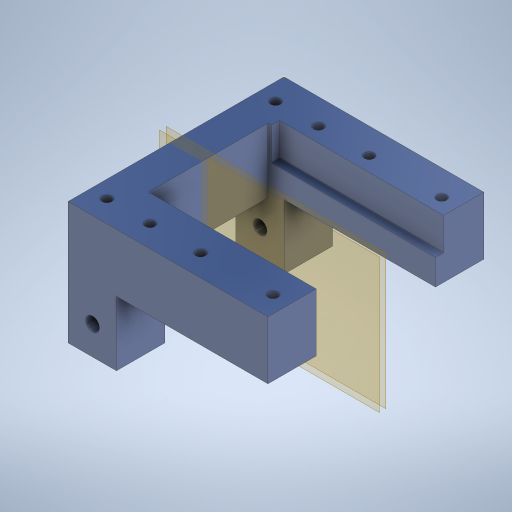
# Autodesk Inventor part: кроншейн
Saved by Autodesk Inventor 2023 (Build 270158000, 158)
## iProperties
Created: 2024-03-12
Part Number: кроншейн
Material: Типовые
Document SubType Name: Modeling
Designer: liza
Density: 1 g/cm^3
Appearance: По умолчанию
Author: liza
Autodesk Inventor part; units mm, degrees
ref_plane "YZ Plane" through (0, 0, 0) normal (1, 0, 0) x (0, 1, 0)
ref_plane "XZ Plane" through (0, 0, 0) normal (0, 1, 0) x (-1, 0, 0)
ref_plane "XY Plane" through (0, 0, 0) normal (0, 0, 1) x (1, 0, 0)
sketch "Эскиз1" plane through (0, 0, 0) normal (0, 0, 1) x (1, 0, 0)
  line L0 (62, -18) -> (62, 0)
  line L1 (62, 0) -> (0, 0)
  line L2 (62, 0) -> (0, 0)
  line L3 (62, -18) -> (15, -18)
  line L4 (0, 0) -> (0, -38)
  line L5 (0, -38) -> (15, -38)
  line L6 (15, -38) -> (15, -18)
  dimension "d27" = 18
  dimension "d32" = 62
  dimension "d40" = 20
  dimension "d41" = 15
  dimension "d42" = 38
  constraints: 14 end point, 2 horizontal, 2 perpendicular, 1 vertical
  measures "d27" distance of L0.start L0.end
  measures "d32" distance of L0.end L1.end
  measures "d40" distance of L3.end L5.end
  measures "d41" distance of L4.end L5.end
  measures "d42" distance of L1.end L4.end
extrude "Выдавливание1" add sketch "Эскиз1" along normal blind 15
sketch "Эскиз2" plane through (0, 0, 0) normal (0, 0, -1) x (-1, 0, 0)
  circle A0 centre (-7.6337, -29.0677) radius 2.1
  point P0 (0, 0)
  dimension "d37" = 4.2
  constraints: 1 centre point
  measures "d37" diameter of A0
extrude "Выдавливание2" cut sketch "Эскиз2" against normal through all
sketch "Эскиз3" plane through (0, 0, 15) normal (0, 0, 1) x (1, 0, 0)
  line L0 (62, 0) -> (0, 0) projected
  line L1 (0, 0) -> (10, 0)
  line L2 (10, 0) -> (10, -20)
  line L3 (10, -20) -> (0, -20)
  line L4 (0, -20) -> (0, 0)
  point P0 (10, 0)
  dimension "d7" = 20
  dimension "d8" = 10
  constraints: 8 end point, 2 parallel, 1 horizontal, 1 perpendicular
  measures "d7" distance of L1.end L2.end
  measures "d8" distance of L2.end L3.end
extrude "Выдавливание3" add sketch "Эскиз3" along normal blind 18.5
mirror "Зеркальное отражение1" about plane through (5, -10, 33.5) normal (0, 0, 1)
sketch "Эскиз6" plane through (0, 0, 0) normal (0, 1, 0) x (1, 0, 0)
  circle A0 centre (5.333, -60.2954) radius 1.5
  circle A1 centre (18.6772, -7.9811) radius 1.5
  circle A2 centre (18.6772, -60.2954) radius 1.5
  circle A3 centre (5.333, -7.9811) radius 1.5
  circle A4 centre (34.4058, -60.2954) radius 1.5
  circle A5 centre (34.4058, -7.9811) radius 1.5
  circle A6 centre (56.8865, -7.9811) radius 1.5
  circle A7 centre (56.8865, -60.2954) radius 1.5
  point P0 (0, 0)
  dimension "d21" = 3
  dimension "d22" = 3
  dimension "d23" = 3
  dimension "d24" = 3
  dimension "d33" = 3
  dimension "d34" = 3
  dimension "d35" = 3
  dimension "d36" = 3
  constraints: 8 centre point
  measures "d21" diameter of A0
  measures "d22" diameter of A1
  measures "d23" diameter of A2
  measures "d24" diameter of A3
  measures "d33" diameter of A4
  measures "d34" diameter of A5
  measures "d35" diameter of A6
  measures "d36" diameter of A7
extrude "Выдавливание6" cut sketch "Эскиз6" against normal blind 13
sketch "Эскиз7" plane through (0, 0, 0) normal (0, 1, 0) x (1, 0, 0)
  line L0 (62, 0) -> (62, -15) projected
  line L1 (62, -15) -> (62, -12.4939)
  line L2 (11.1046, -12.4939) -> (11.1046, -15)
  line L3 (62, -15) -> (10, -15) projected
  line L4 (62, -15) -> (11.1046, -15)
  line L5 (11.1046, -12.4939) -> (62, -12.4939)
  point P0 (0, 0)
  constraints: 8 end point, 2 parallel, 2 point on line, 1 perpendicular
extrude "Выдавливание7" cut sketch "Эскиз7" against normal blind 10
sketch "Эскиз8" plane through (0, -38, 0) normal (-1, 0, 0) x (0, 0, 1)
  point P0 (0, 38)
ref_plane "РабПлоскость3" through (0, 0, 35.5) normal (0, 0, 1) x (1, 0, 0)
ref_plane "РабПлоскость2" through (0, 0, 33.5) normal (0, 0, 1) x (1, 0, 0)
sketch "Эскиз9" plane through (0, 0, 35.5) normal (0, 0, 1) x (1, 0, 0)
  line L0 (0, 0) -> (0, -38) projected
  circle A0 centre (-10.4982, -19.8582) radius 5
  line L1 (0, -20) -> (0, -38) projected
  line L2 (0, -14.2319) -> (0, -12.6158)
  circle A1 centre (-10.4982, -19.8582) radius 2.1
  line L3 (0, -12.6158) -> (0, -14.2319)
  line L4 (-13.4667, -15.8348) -> (1.5377, -4.7644)
  line L5 (-6.9627, -23.3937) -> (0, -16.431)
  line L6 (0, -5.899) -> (0, -16.431)
  point P0 (-15.4732, -20.3581)
  point P1 (-12.5479, -24.4188)
  point P2 (0, -3.6635)
  dimension "d46" = 4.2
  dimension "d47" = 10
  dimension "d52" = 45
  constraints: 10 end point, 4 point on circle, 3 vertical, 2 centre point, 2 point on line, 2 tangent, 1 coincident, 5 other
  measures "d46" diameter of A1
  measures "d47" diameter of A0
  measures "d52" angle to the sketch x axis of L5
extrude "Выдавливание8" add sketch "Эскиз9" along normal blind 4
mirror "Зеркальное отражение2" about plane through (0, 0, 33.5) normal (0, 0, 1) of "Выдавливание8"
